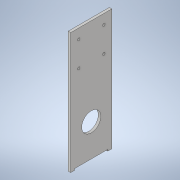
# Autodesk Inventor part: center wall
Saved by Autodesk Inventor 2020 (Build 240168000, 168)
## iProperties
Created: 2018-12-12
Part Number: center wall
Material: Generic
Document SubType Name: Modeling
Designer: aonih
Density: 1 g/cm^3
Appearance: Default
Author: aonih
Autodesk Inventor part; units mm, degrees
ref_plane "YZ Plane" through (0, 0, 0) normal (1, 0, 0) x (0, 1, 0)
ref_plane "XZ Plane" through (0, 0, 0) normal (0, 1, 0) x (-1, 0, 0)
ref_plane "XY Plane" through (0, 0, 0) normal (0, 0, 1) x (1, 0, 0)
sketch "Sketch1" plane through (0, 0, 0) normal (1, 0, 0) x (0, 1, 0)
  line L0 (128.3979, 81.9005) -> (-112.6021, 81.9005)
  line L1 (-112.6021, 81.9005) -> (-112.6021, -0.0995)
  line L2 (-112.6021, -0.0995) -> (128.3979, -0.0995)
  line L3 (128.3979, -0.0995) -> (128.3979, 81.9005)
  circle A0 centre (-45.6021, 40.9005) radius 19
  line L4 (-112.6021, 73.9005) -> (-109.6021, 73.9005)
  line L5 (-109.6021, 73.9005) -> (-109.6021, 7.9005)
  line L6 (-109.6021, 7.9005) -> (-112.6021, 7.9005)
  line L7 (-112.6021, 7.9005) -> (-112.6021, 73.9005)
  point P0 (0, 0)
  dimension "d0" = 241
  dimension "d1" = 82
  dimension "d2" = 38
  dimension "d3" = 41
  dimension "d4" = 174
  dimension "d5" = 66
  dimension "d6" = 3
  dimension "d7" = 8
  constraints: 16 end point, 4 parallel, 2 horizontal, 2 perpendicular, 1 centre point, 1 point on line
  measures "d0" distance of L1.end L2.end
  measures "d1" distance of L2.end L0.start
  measures "d2" diameter of A0
  measures "d3" distance from line of L0 A0.centre
  measures "d4" distance from line of L3 A0.centre
  measures "d5" distance of L4.end L5.end
  measures "d6" distance of L5.end L6.end
  measures "d7" distance from line of L2 L5.end
extrude "Extrusion1" add sketch "Sketch1" along normal blind 5 contours L3 L2 L1 L6 L5 L4 L0
sketch "Sketch2" plane through (5, 0, 0) normal (1, 0, 0) x (0, 0, -1)
  circle A0 centre (-40.9005, -45.6021) radius 19 projected
  circle A1 centre (-65.9005, 108.8979) radius 2.5
  line L0 (-81.9005, 128.3979) -> (-81.9005, -112.6021) construction
  line L1 (0.0995, 128.3979) -> (-81.9005, 128.3979) construction
  line L2 (-81.9005, 128.3979) -> (0.0995, 128.3979) construction
  line L3 (-81.9005, 128.3979) -> (-81.9005, -112.6021) construction
  circle A2 centre (-15.9005, 108.8979) radius 2.5
  circle A3 centre (-65.9005, 58.8979) radius 2.5
  circle A4 centre (-15.9005, 58.8979) radius 2.5
  line L4 (-65.9005, 58.8979) -> (-15.9005, 58.8979) construction
  line L5 (-15.9005, 58.8979) -> (-15.9005, 108.8979) construction
  point P0 (0, 0)
  point P1 (-40.9005, 58.8979)
  dimension "d10" = 5
  dimension "d13" = 50
  dimension "d16" = 50
  dimension "d19" = 19.5
  constraints: 8 end point, 4 centre point, 2 collinear, 2 horizontal, 1 coincident, 1 midpoint, 1 perpendicular, 1 vertical, 1 vertical alignment, 6 other
  measures "d10" diameter of A1
  measures "d13" distance of A1.centre L5.end
  measures "d16" distance of A1.centre L4.start
  measures "d19" distance from line of L1 A1.centre
extrude "Extrusion2" cut sketch "Sketch2" against normal up to surface (5 mm away) contours A1 | A2 | A3 | A4
equation "\"d3\" = 0.5 * d1"
equation "\"d7\" = -0.5 * d5 + 0.5 * d1"
body "Solid1"
